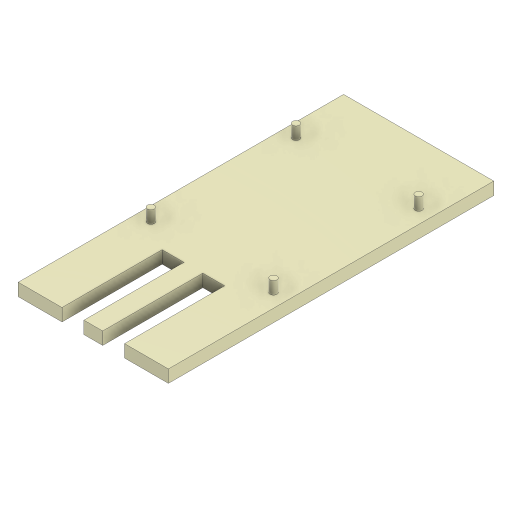
# Autodesk Inventor part: Platform
Saved by Autodesk Inventor 2023.4 (Build 274418000, 418)
## iProperties
Created: 2024-02-27
Part Number: Platform
Material: Generic
Document SubType Name: Modeling
Designer: josep
Density: 1 g/cm^3
Appearance: Default
Author: josep
Autodesk Inventor part; units mm, degrees
ref_plane "YZ Plane" through (0, 0, 0) normal (1, 0, 0) x (0, 1, 0)
ref_plane "XZ Plane" through (0, 0, 0) normal (0, 1, 0) x (-1, 0, 0)
ref_plane "XY Plane" through (0, 0, 0) normal (0, 0, 1) x (1, 0, 0)
sketch "Sketch1" plane through (0, 0, 0) normal (0, 1, 0) x (-1, 0, 0)
  line L0 (30, 45) -> (-30, 45)
  line L1 (-30, 45) -> (-30, -45)
  line L2 (-30, -45) -> (30, -45)
  line L3 (30, -45) -> (30, 45)
  line L4 (30, 45) -> (12.5, 45)
  line L5 (12.5, 45) -> (12.5, 85)
  line L6 (12.5, 85) -> (30, 85)
  line L7 (30, 85) -> (30, 45)
  line L8 (-30, 45) -> (-12.5, 45)
  line L9 (-12.5, 45) -> (-12.5, 85)
  line L10 (-12.5, 85) -> (-30, 85)
  line L11 (-30, 85) -> (-30, 45)
  line L12 (3.75, 45) -> (-3.75, 45)
  line L13 (-3.75, 45) -> (-3.75, 85)
  line L14 (-3.75, 85) -> (3.75, 85)
  line L15 (3.75, 85) -> (3.75, 45)
  point P0 (0, 0)
  point P1 (0, 45)
  dimension "d0" = 90
  dimension "d1" = 60
  dimension "d2" = 45
  dimension "d3" = 30
  dimension "d23" = 40
  dimension "d24" = 25
  dimension "d25" = 17.5
  dimension "d39" = 7.5
  dimension "d40" = 40
  dimension "d41" = 3.75
  constraints: 32 end point, 8 parallel, 4 horizontal, 4 perpendicular, 2 point on line, 1 midpoint
  measures "d0" distance of L2.end L0.start
  measures "d1" distance of L1.end L2.end
  measures "d2" vertical distance of L0.start point (0, 0)
  measures "d3" horizontal distance of point (0, 0) L1.end
  measures "d23" distance of L6.end L0.start
  measures "d24" distance of L8.end L4.end
  measures "d25" distance of L8.end L0.end
  measures "d39" distance of L13.end L14.end
  measures "d40" distance of L14.end L12.start
  measures "d41" distance of L12.end point (0, 45)
extrude "Extrusion1" add sketch "Sketch1" along normal blind 5
sketch "Sketch2" plane through (0, 5, 0) normal (0, 1, 0) x (1, 0, 0)
  line L0 (-24.5, -37.5) -> (24.5, -37.5)
  line L1 (24.5, -37.5) -> (24.5, 20.5)
  line L2 (24.5, 20.5) -> (-24.5, 20.5)
  line L3 (-24.5, 20.5) -> (-24.5, -37.5)
  line L4 (-12.5, -45) -> (12.5, -45) projected
  circle A0 centre (-24.5, -37.5) radius 1.35
  line L5 (-24.5, -8.5) -> (24.5, -8.5)
  line L6 (0, -37.5) -> (0, 20.5)
  circle A1 centre (24.5, -37.5) radius 1.35
  circle A2 centre (-24.5, 20.5) radius 1.35
  circle A3 centre (24.5, 20.5) radius 1.35
  point P0 (0, 0)
  point P1 (-30, -45)
  point P2 (30, -45)
  dimension "d6" = 49
  dimension "d7" = 58
  dimension "d8" = 24.5
  dimension "d9" = 7.5
  dimension "d10" = 2.7
  dimension "d13" = 49
  dimension "d16" = 58
  constraints: 12 end point, 4 centre point, 4 midpoint, 2 horizontal, 2 parallel, 1 coincident, 1 perpendicular, 1 vertical, 6 other
  measures "d6" distance of L0.start L0.end
  measures "d7" distance of L2.end L0.start
  measures "d8" horizontal distance of L0.end point (0, 0)
  measures "d9" distance between parallel lines of L4 L0
  measures "d10" diameter of A0
  measures "d13" distance of A0.centre A1.centre
  measures "d16" distance of A0.centre A2.centre
extrude "Extrusion2" add sketch "Sketch2" along normal blind 5 contours L3 A0 L0 | L0 A0 L3 | A1 L1 L0 | L0 L1 A1 | A2 L2 L3 | L3 L2 A2 | A3 L2 L1 | L1 L2 A3
sketch "Sketch4" plane through (0, 0, 0) normal (1, 0, 0) x (0, 1, 0)
  line L0 (0, -45) -> (5, -45) projected
  line L1 (0, -45) -> (-16.853, -30.8587)
  line L2 (-16.853, -30.8587) -> (-15.246, -28.9436)
  line L3 (-15.246, -28.9436) -> (0, -41.7365)
  line L4 (0, -45) -> (0, 85) projected
  point P0 (0, 0)
  dimension "d28" = 130
  dimension "d29" = 2.5
  dimension "d30" = 22
  constraints: 6 end point, 1 parallel, 1 perpendicular, 1 point on line
  measures "d28" angle of L4 L1
  measures "d29" distance of L1.end L2.end
  measures "d30" distance of L0.start L1.end
extrude "Extrusion4" add sketch "Sketch4" along normal mid plane 25
sketch "Sketch6" plane through (12.5, 0, -45) normal (0, -0.6428, -0.766) x (-1, 0, 0)
  line L0 (-17.5, 0) -> (0, 0) projected
  line L1 (25, -22) -> (0, -22) projected
  line L2 (0, 0) -> (25, 0)
  line L3 (25, 0) -> (25, -22)
  line L4 (25, -22) -> (0, -22)
  line L5 (0, -22) -> (0, 0)
  line L6 (25, -2.0977) -> (0, -2.0977) projected
  circle A0 centre (2, -5.638) radius 1.1
  circle A1 centre (23, -5.638) radius 1.1
  circle A2 centre (2, -18.138) radius 1.1
  circle A3 centre (23, -18.138) radius 1.1
  line L7 (8.25, -13.788) -> (16.75, -13.788)
  line L8 (16.75, -13.788) -> (16.75, -22.288)
  line L9 (16.75, -22.288) -> (8.25, -22.288)
  line L10 (8.25, -22.288) -> (8.25, -13.788)
  line L11 (0, -22) -> (0, 0) projected
  line L12 (25, -22) -> (25, -2.0977) projected
  line L13 (0, -3.638) -> (25, -3.638)
  line L14 (25, -3.638) -> (25, -27.5)
  line L15 (25, -27.5) -> (0, -27.5)
  line L16 (0, -27.5) -> (0, -3.638)
  line L17 (12.5, -13.788) -> (12.5, -22.288)
  line L18 (8.25, -18.038) -> (16.75, -18.038)
  dimension "d42" = 2.2
  dimension "d43" = 2.2
  dimension "d44" = 2.2
  dimension "d45" = 2.2
  dimension "d47" = 2
  dimension "d48" = 0
  dimension "d50" = 0
  dimension "d52" = 0
  dimension "d53" = 2
  dimension "d56" = 0
  dimension "d59" = 12.5
  dimension "d60" = 8.5
  dimension "d61" = 8.5
  dimension "d63" = 23.862
  dimension "d65" = 2
  dimension "d66" = 12.5
  dimension "d69" = 9.462
  dimension "d70" = 5.5
  constraints: 28 end point, 6 parallel, 4 centre point, 4 midpoint, 4 perpendicular, 3 horizontal, 2 point on line
  measures "d42" diameter of A0
  measures "d43" diameter of A2
  measures "d44" diameter of A3
  measures "d45" diameter of A1
  measures "d47" distance from line of L5 A0.centre
  measures "d48" horizontal distance of A0.centre A2.centre
  measures "d50" horizontal distance of A3.centre A1.centre
  measures "d52" vertical distance of A0.centre A1.centre
  measures "d53" distance from line of L3 A1.centre
  measures "d56" vertical distance of A3.centre A2.centre
  measures "d59" distance from line of L5 L17.start
  measures "d60" distance of L7.end L8.end
  measures "d61" distance of L7.start L7.end
  measures "d63" distance of L15.end L13.start
  measures "d65" distance from line of L13 A1.centre
  measures "d66" distance of A2.centre A0.centre
  measures "d69" distance from line of L15 L18.end
  measures "d70" distance between parallel lines of L15 L1
extrude "Extrusion5" cut sketch "Sketch6" against normal blind 5 contours A0 | A1 | A2 | A3
sketch "Sketch9" plane through (12.5, 0, -45) normal (0, -0.6428, -0.766) x (-1, 0, 0)
  circle A0 centre (12.5, -18.038) radius 0.2236
  point P0 (12.5, -28.9254)
  constraints: 1 centre point
body "Solid1"
